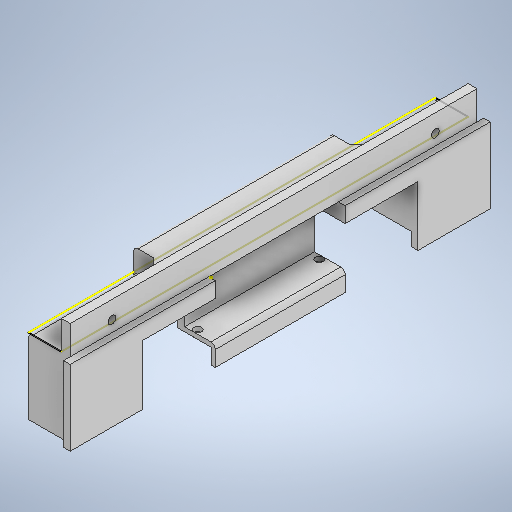
# Autodesk Inventor part: D1-bottom
Saved by Autodesk Inventor 2025.2 (Build 292293000, 293)
## iProperties
Created: 2025-11-15
Part Number: D1-bottom
Material: 일반
Document SubType Name: Modeling
Designer: RunGeun
Density: 1 g/cm^3
Appearance: 기본값
Author: RunGeun
Autodesk Inventor part; units mm, degrees
ref_plane "YZ Plane" through (0, 0, 0) normal (1, 0, 0) x (0, 1, 0)
ref_plane "XZ Plane" through (0, 0, 0) normal (0, 1, 0) x (-1, 0, 0)
ref_plane "XY Plane" through (0, 0, 0) normal (0, 0, 1) x (1, 0, 0)
sketch "스케치1" plane through (0, 0, 0) normal (0, 1, 0) x (-1, 0, 0)
  line L0 (0, 0) -> (15.1, 0)
  line L1 (15.1, 0) -> (15.1, -58.7)
  line L2 (15.1, -58.7) -> (0, -58.7)
  line L3 (0, -58.7) -> (0, 0)
  circle A0 centre (8, -1.85) radius 1.75
  circle A1 centre (8, -56.85) radius 1.75
  line L4 (15.1, 0) -> (12.1, 0)
  line L5 (12.1, 0) -> (12.1, -58.7)
  line L6 (12.1, -58.7) -> (15.1, -58.7)
  line L7 (15.1, -58.7) -> (15.1, 0)
  line L8 (0, 0) -> (-1.8, 0)
  line L9 (-1.8, 0) -> (-1.8, -58.7)
  line L10 (-1.8, -58.7) -> (0, -58.7)
  line L11 (0, -58.7) -> (0, 0)
  point P0 (0, -58.7)
  dimension "d0" = 58.7
  dimension "d1" = 15.1
  dimension "d2" = 8
  dimension "d3" = 3.5
  dimension "d4" = 3.5
  dimension "d5" = 8
  dimension "d6" = 3
  dimension "d11" = 1.8
  dimension "d15" = 1.85
  dimension "d16" = 1.85
  constraints: 24 end point, 6 parallel, 3 horizontal, 3 perpendicular, 2 centre point, 1 point on line
  measures "d0" distance of L2.end L0.start
  measures "d1" distance of L1.end L2.end
  measures "d2" distance from line of A0.centre L3
  measures "d3" diameter of A0
  measures "d4" diameter of A1
  measures "d5" distance from line of A1.centre L3
  measures "d6" distance between parallel lines of L1 L5
  measures "d11" distance of L9.end L10.end
  measures "d15" distance from line of A0.centre L0
  measures "d16" distance from line of A1.centre L2
extrude "돌출1" add sketch "스케치1" along normal blind 20 contours L0 L1 L2 L5
extrude "돌출2" add sketch "스케치1" along normal blind 2 contours L0 L5 L2 L3 | L3 L10 L9 L8
sketch "스케치2" plane through (0, 0, 0) normal (0, -1, 0) x (1, 0, 0)
  line L0 (-15.1, 0) -> (1.8, 0) projected
  line L1 (1.8, -58.7) -> (-15.1, -58.7) projected
  line L2 (1.8, 0) -> (0, 0)
  line L3 (0, 0) -> (0, -58.7)
  line L4 (0, -58.7) -> (1.8, -58.7)
  line L5 (1.8, -58.7) -> (1.8, 0)
  point P0 (0, 0)
  dimension "d12" = 1.8
  constraints: 8 end point, 2 parallel, 1 horizontal, 1 perpendicular, 1 point on line
  measures "d12" distance between parallel lines of L5 L3
extrude "돌출3" add sketch "스케치2" along normal blind 7
sketch "스케치3" plane through (0, 20, 0) normal (0, 1, 0) x (1, 0, 0)
  line L0 (1.8, 58.7) -> (-12.1, 58.7) projected
  line L1 (-12.1, 58.7) -> (-20.1, 58.7)
  line L2 (-20.1, 58.7) -> (-20.1, 0)
  line L3 (-20.1, 0) -> (-12.1, 0)
  line L4 (-12.1, 0) -> (-12.1, 58.7)
  line L5 (-20.1, 0) -> (1.8, 0)
  line L6 (1.8, 0) -> (1.8, -32.9)
  line L7 (1.8, -32.9) -> (-20.1, -32.9)
  line L8 (-20.1, -32.9) -> (-20.1, 0)
  line L9 (-20.1, 58.7) -> (1.8, 58.7)
  line L10 (1.8, 58.7) -> (1.8, 91.6)
  line L11 (1.8, 91.6) -> (-20.1, 91.6)
  line L12 (-20.1, 91.6) -> (-20.1, 58.7)
  line L13 (-12.1, 0) -> (1.8, 0) projected
  line L14 (1.8, 0) -> (1.8, 58.7) projected
  line L15 (1.8, -32.9) -> (-20.1, -32.9)
  line L16 (-20.1, -32.9) -> (-20.1, -65.6)
  line L17 (-20.1, -65.6) -> (1.8, -65.6)
  line L18 (1.8, -65.6) -> (1.8, -32.9)
  line L19 (-20.1, 91.6) -> (1.8, 91.6)
  line L20 (1.8, 91.6) -> (1.8, 124.3)
  line L21 (1.8, 124.3) -> (-20.1, 124.3)
  line L22 (-20.1, 124.3) -> (-20.1, 91.6)
  point P0 (0, 0)
  dimension "d17" = 8
  dimension "d18" = 32.9
  dimension "d19" = 32.9
  dimension "d20" = 0
  dimension "d21" = 0
  dimension "d24" = 32.7
  dimension "d25" = 32.7
  constraints: 40 end point, 10 parallel, 5 horizontal, 5 perpendicular, 2 point on line
  measures "d17" distance between parallel lines of L4 L2
  measures "d18" distance between parallel lines of L0 L11
  measures "d19" distance of L5.end L6.end
  measures "d20" distance between parallel lines of L13 L5
  measures "d21" distance between parallel lines of L14 L6
  measures "d24" distance of L16.end L15.end
  measures "d25" distance of L19.end L20.end
extrude "돌출4" add sketch "스케치3" along normal blind 7 contours L0 L1 L12 L11 L10 | L4 L3 L2 L1 | L11 L22 L21 L20 | L6 L7 L8 L3 L5 | L18 L17 L16 L7
extrude "돌출5" add sketch "스케치3" against normal blind 27 contours L11 L22 L21 L20 | L18 L17 L16 L7
sketch "스케치4" plane through (0, -7, 0) normal (0, -1, 0) x (1, 0, 0)
  line L0 (-1, 49.5) -> (-7, 49.5)
  line L1 (-7, 49.5) -> (-7, 34.2)
  line L2 (-7, 34.2) -> (-1, 34.2)
  line L3 (-1, 34.2) -> (-1, 49.5)
  line L4 (-1, -92.9) -> (-7, -92.9)
  line L5 (-7, -92.9) -> (-7, -108.2)
  line L6 (-7, -108.2) -> (-1, -108.2)
  line L7 (-1, -108.2) -> (-1, -92.9)
  line L8 (-20.1, 32.9) -> (1.8, 32.9) projected
  line L9 (1.8, -91.6) -> (-20.1, -91.6) projected
  line L10 (1.8, 32.9) -> (1.8, 65.6) projected
  line L11 (1.8, -124.3) -> (1.8, -91.6) projected
  point P0 (0, 0)
  dimension "d28" = 15.3
  dimension "d29" = 15.3
  dimension "d30" = 6
  dimension "d31" = 6
  dimension "d32" = 1.3
  dimension "d33" = 1.3
  dimension "d34" = 2.8
  dimension "d35" = 2.8
  constraints: 16 end point, 4 parallel, 2 horizontal, 2 perpendicular
  measures "d28" distance of L0.end L1.end
  measures "d29" distance of L4.end L5.end
  measures "d30" distance of L5.end L6.end
  measures "d31" distance of L1.end L2.end
  measures "d32" distance between parallel lines of L8 L2
  measures "d33" distance between parallel lines of L9 L4
  measures "d34" distance between parallel lines of L10 L3
  measures "d35" distance between parallel lines of L11 L7
extrude "돌출6" cut sketch "스케치4" against normal blind 23
sketch "스케치5" plane through (1.8, 27, -124.3) normal (0, 0, -1) x (-1, 0, 0)
  line L0 (0, -34) -> (21.9, -34) projected
  line L1 (21.9, 0) -> (0, 0) projected
  line L2 (0, -34) -> (21.9, -34)
  line L3 (21.9, -34) -> (21.9, 0)
  line L4 (21.9, 0) -> (0, 0)
  line L5 (0, 0) -> (0, -34)
  line L6 (0, 0) -> (3, 0)
  line L7 (3, 0) -> (3, -34)
  line L8 (3, -34) -> (0, -34)
  line L9 (0, -34) -> (0, 0)
  point P0 (1.8, -27)
  dimension "d38" = 3
  constraints: 16 end point, 4 parallel, 2 horizontal, 2 perpendicular, 1 point on line
  measures "d38" distance of L7.end L8.end
extrude "돌출7" cut sketch "스케치5" against normal blind 3 contours L7 L1 L3 L0
sketch "스케치6" plane through (-20.1, 27, 65.6) normal (0, 0, 1) x (1, 0, 0)
  line L0 (18.9, 0) -> (0, 0) projected
  line L1 (21.9, -34) -> (21.9, 0) projected
  line L2 (0, 0) -> (21.9, 0)
  line L3 (21.9, 0) -> (21.9, -34)
  line L4 (21.9, -34) -> (0, -34)
  line L5 (0, -34) -> (0, 0)
  line L6 (8, 0) -> (21.9, 0) projected
  line L7 (21.9, -34) -> (18.9, -34)
  line L8 (18.9, -34) -> (18.9, 0)
  line L9 (18.9, 0) -> (21.9, 0)
  line L10 (21.9, 0) -> (21.9, -34)
  point P0 (20.1, -27)
  point P1 (18.9, 0)
  dimension "d41" = 3
  constraints: 16 end point, 4 parallel, 2 horizontal, 2 perpendicular, 1 point on line
  measures "d41" distance of L8.end L9.end
extrude "돌출8" cut sketch "스케치6" against normal blind 3 contours L8 L4 L5 L0
sketch "스케치7" plane through (0, 27, 0) normal (0, 1, 0) x (1, 0, 0)
  line L0 (-1.2, -62.6) -> (-1.2, -65.6) projected
  line L1 (-1.2, 121.3) -> (-20.1, 121.3) projected
  line L2 (-1.2, -62.6) -> (-5.2, -62.6)
  line L3 (-5.2, -62.6) -> (-5.2, 121.3)
  line L4 (-5.2, 121.3) -> (-1.2, 121.3)
  line L5 (-1.2, 121.3) -> (-1.2, -62.6)
  point P0 (0, 0)
  dimension "d44" = 4
  constraints: 8 end point, 2 parallel, 1 horizontal, 1 perpendicular, 1 point on line
  measures "d44" distance of L3.end L4.end
extrude "돌출9" add sketch "스케치7" along normal blind 13
sketch "스케치8" plane through (0, 27, 0) normal (0, 1, 0) x (1, 0, 0)
  line L0 (-5.2, 121.3) -> (-5.2, -62.6) projected
  line L1 (-20.1, 121.3) -> (-20.1, -62.6) projected
  line L2 (-5.2, -62.6) -> (-20.1, -62.6)
  line L3 (-20.1, -62.6) -> (-20.1, 121.3)
  line L4 (-20.1, 121.3) -> (-5.2, 121.3)
  line L5 (-5.2, 121.3) -> (-5.2, -62.6)
  point P0 (0, 0)
  constraints: 8 end point, 2 parallel, 1 horizontal, 1 perpendicular
sketch "스케치9" plane through (-1.2, 27, 0) normal (1, 0, 0) x (0, 0, -1)
  circle A0 centre (-43.75, 5) radius 1.75
  circle A1 centre (102.45, 5) radius 1.75
  line L0 (-65.6, 0) -> (0, 0) projected
  line L1 (58.7, 0) -> (124.3, 0) projected
  line L2 (-62.6, 0) -> (-62.6, 13) projected
  line L3 (-65.6, -34) -> (-65.6, 0) projected
  line L4 (124.3, -34) -> (124.3, 0) projected
  point P0 (0, -27)
  dimension "d47" = 3.5
  dimension "d48" = 3.5
  dimension "d49" = 5
  dimension "d50" = 5
  dimension "d52" = 21.85
  dimension "d53" = 21.85
  constraints: 2 centre point
  measures "d47" diameter of A1
  measures "d48" diameter of A0
  measures "d49" distance from line of A0.centre L0
  measures "d50" distance from line of A1.centre L1
  measures "d52" distance from line of A0.centre L3
  measures "d53" distance from line of A1.centre L4
extrude "돌출10" cut sketch "스케치9" against normal blind 10
sketch "스케치10" plane through (0, 27, 0) normal (0, 1, 0) x (1, 0, 0)
  line L0 (-20.1, 91.6) -> (-20.1, -32.9) projected
  line L1 (-5.2, -62.6) -> (-5.2, 0) projected
  line L2 (-20.1, 73.7) -> (-5.2, 73.7)
  line L3 (-5.2, 73.7) -> (-5.2, -15)
  line L4 (-5.2, -15) -> (-20.1, -15)
  line L5 (-20.1, -15) -> (-20.1, 73.7)
  line L6 (-5.2, 0) -> (-12.1, 0) projected
  line L7 (-12.1, 58.7) -> (-5.2, 58.7) projected
  point P0 (0, 0)
  dimension "d56" = 15
  dimension "d57" = 15
  constraints: 8 end point, 2 parallel, 2 point on line, 1 horizontal, 1 perpendicular
  measures "d56" distance between parallel lines of L6 L4
  measures "d57" distance between parallel lines of L7 L2
extrude "돌출11" add sketch "스케치10" along normal blind 10
chamfer "모따기1" distance 6 angle 45 2 edges at (-5.2, 32, -73.7) (-5.2, 32, 15)
fillet "모깎기1" radius 2 5 edges at (-12.1, 27, -29.35) (-20.1, 37, -29.35) (-20.1, 27, -97.5) (-20.1, 27, 38.8) (1.8, 2, -29.35)
sketch "스케치11" plane through (0, -7, 0) normal (0, -1, 0) x (1, 0, 0)
  line L0 (-20.1, 32.9) -> (1.8, 32.9) projected
  line L1 (-1, 49.5) -> (-1, 34.2) projected
  line L2 (-20.1, 32.9) -> (-1, 32.9)
  line L3 (-1, 32.9) -> (-1, 52.9)
  line L4 (-1, 52.9) -> (-20.1, 52.9)
  line L5 (-20.1, 52.9) -> (-20.1, 32.9)
  line L6 (-1, -92.9) -> (-1, -108.2) projected
  line L7 (-20.1, -91.6) -> (-1, -91.6)
  line L8 (-1, -91.6) -> (-1, -111.6)
  line L9 (-1, -111.6) -> (-20.1, -111.6)
  line L10 (-20.1, -111.6) -> (-20.1, -91.6)
  point P0 (0, 0)
  point P1 (-1, 32.9)
  dimension "d64" = 20
  dimension "d65" = 20
  constraints: 16 end point, 4 parallel, 2 horizontal, 2 perpendicular, 2 point on line
  measures "d64" distance between parallel lines of L0 L4
  measures "d65" distance between parallel lines of L7 L9
extrude "돌출12" cut sketch "스케치11" against normal blind 6
equation "\"d4\" = d3"
equation "\"d5\" = d2"
equation "\"d16\" = d15"
equation "\"d18\" = d19"
equation "\"d25\" = d24"
equation "\"d29\" = d28"
equation "\"d31\" = d30"
equation "\"d32\" = d33"
equation "\"d35\" = d34"
equation "\"d50\" = d49"
equation "\"d53\" = d52"
equation "\"d65\" = d64"
